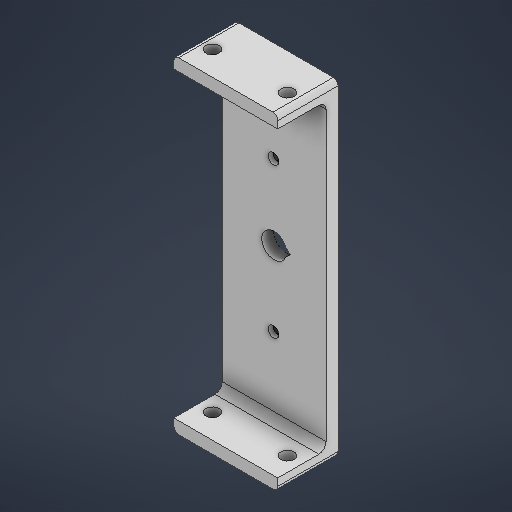
# Autodesk Inventor part: motor_holder
Saved by Autodesk Inventor 2026 (Build 300175050, 175E)
## iProperties
Created: 2025-01-16
Part Number: motor_holder
Material: Generic
Document SubType Name: Modeling
Designer: aduwa
Density: 1 g/cm^3
Appearance: Default
Author: aduwa
Autodesk Inventor part; units mm, degrees
ref_plane "YZ Plane" through (0, 0, 0) normal (1, 0, 0) x (0, 1, 0)
ref_plane "XZ Plane" through (0, 0, 0) normal (0, 1, 0) x (-1, 0, 0)
ref_plane "XY Plane" through (0, 0, 0) normal (0, 0, 1) x (1, 0, 0)
sketch "Sketch1" plane through (0, 0, 0) normal (0, 0, 1) x (1, 0, 0)
  circle A0 centre (0, 0) radius 2.25
  circle A1 centre (31, 0) radius 2.25
  circle A2 centre (0, 31) radius 2.25
  circle A3 centre (31, 31) radius 2.25
  circle A4 centre (15.5, 15.5) radius 5.125
  line L0 (-6, 37) -> (37, 37)
  line L1 (37, 37) -> (37, -6)
  line L2 (37, -6) -> (-6, -6)
  line L3 (-6, -6) -> (-6, 37)
  line L4 (-6, 37) -> (37, -6) construction
  line L5 (37, 37) -> (-6, -6) construction
  line L6 (-6, -6) -> (37, -6)
  line L7 (37, -6) -> (37, -52)
  line L8 (37, -52) -> (-6, -52)
  line L9 (-6, -52) -> (-6, -6)
  line L10 (-6, 15.5) -> (0, 15.5)
  line L11 (37, 37) -> (37, 83)
  line L12 (37, 83) -> (-6, 83)
  line L13 (-6, 83) -> (-6, 37)
  line L14 (20.625, 15.5) -> (22.125, 15.5)
  line L15 (22.125, 15.5) -> (20.2868, 17.3309)
  line L16 (22.125, 15.5) -> (20.2868, 13.6691)
  point P0 (37, 37)
  dimension "d3" = 4.5
  dimension "d5" = 31
  dimension "d6" = 10.25
  dimension "d7" = 43
  dimension "d8" = 43
  dimension "d9" = 67.5
  dimension "d10" = 31
  dimension "d44" = 1.5
  constraints: 34 end point, 5 centre point, 4 horizontal, 4 parallel, 3 equal radius, 3 midpoint, 3 point on circle, 3 symmetric about line, 2 perpendicular, 2 vertical alignment, 1 horizontal alignment
  measures "d3" diameter of A0
  measures "d5" distance of A0.centre A2.centre
  measures "d6" diameter of A4
  measures "d7" distance of L1.end L2.end
  measures "d8" distance of L0.end L1.end
  measures "d9" distance from line of L8 A4.centre
  measures "d10" distance of A3.centre A2.centre
  measures "d44" distance of L14.start L14.end
extrude "Extrusion1" add sketch "Sketch1" against normal blind 5 contours A0 | A1 | A2 | A3 | L13 L12 L11 L0 | L0 L1 L2 L3 | L7 L8 L9 L2
sketch "Sketch2" plane through (0, 0, 0) normal (0, 0, 1) x (1, 0, 0)
  line L0 (37, -52) -> (-6, -52) projected
  line L1 (37, 83) -> (37, -52) projected
  line L2 (-6, -52) -> (37, -52)
  line L3 (37, -52) -> (37, -47)
  line L4 (37, -47) -> (-6, -47)
  line L5 (-6, -47) -> (-6, -52)
  line L6 (-6, 15.5) -> (0, 15.5) projected
  line L7 (37, 78) -> (-6, 78)
  line L8 (-6, 78) -> (37, 78)
  line L9 (-6, 83) -> (-6, -52) projected
  line L10 (-6, -52) -> (37, -52) projected
  line L11 (37, -52) -> (37, 83) projected
  line L12 (37, 83) -> (-6, 83) projected
  arc A0 (20.2868, 17.3309) -> (20.2868, 13.6691) centre (15.5, 15.5) ccw projected
  line L13 (22.125, 15.5) -> (20.2868, 13.6691) projected
  line L14 (20.2868, 17.3309) -> (22.125, 15.5) projected
  point P0 (0, 0)
  point P1 (37, 37)
  point P2 (-6, 37)
  point P3 (-6, 78)
  point P4 (37, 78)
  dimension "d13" = 5
  constraints: 12 end point, 3 equal length, 2 symmetric about line, 1 horizontal, 1 perpendicular, 1 point on line
  measures "d13" distance of L3.end L2.end
extrude "Extrusion2" add sketch "Sketch2" along normal blind 20 contours L0 L5 L4 L1 | L7 L9 L12 L1
sketch "Sketch3" plane through (-6, -47, 0) normal (0, 1, 0) x (1, 0, 0)
  circle A0 centre (6, -10) radius 2.75
  circle A1 centre (37, -10) radius 2.75
  line L0 (0, 5) -> (0, -20) projected
  line L1 (0, 0) -> (0, -20) projected
  line L2 (43, 0) -> (43, -20) projected
  line L3 (0, 5) -> (43, 5) projected
  line L4 (0, 0) -> (43, 0) projected
  line L5 (43, 5) -> (0, 5) projected
  line L6 (6, -10) -> (6, -15) construction
  arc A2 (8.75, -10) -> (3.25, -10) centre (6, -10) ccw
  line L7 (21.5, 0) -> (21.5, -10)
  arc A3 (39.75, -10) -> (34.25, -10) centre (37, -10) ccw
  line L8 (6, -10) -> (6, -5) construction
  line L9 (3.25, -10) -> (3.25, -5)
  line L10 (8.75, -5) -> (8.75, -10)
  arc A4 (3.25, -10) -> (8.75, -10) centre (6, -10) ccw
  arc A5 (8.75, -5) -> (3.25, -5) centre (6, -5) ccw
  line L11 (37, -10) -> (37, -5) construction
  line L12 (39.75, -10) -> (39.75, -5)
  line L13 (34.25, -5) -> (34.25, -10)
  arc A6 (39.75, -5) -> (34.25, -5) centre (37, -5) ccw
  point P0 (6, 0)
  point P1 (0, -10)
  point P2 (6, -12.5)
  point P3 (6, -7.5)
  point P4 (39.75, -10)
  point P5 (3.25, -10)
  dimension "d16" = 5.5
  dimension "d17" = 31
  dimension "d23" = 6
  dimension "d38" = 15
  dimension "d39" = 5
  dimension "d43" = 5
  constraints: 22 end point, 10 point on circle, 9 symmetric about line, 7 centre point, 4 midpoint, 4 tangent, 3 equal radius, 3 vertical, 1 horizontal alignment, 1 parallel, 2 other
  measures "d16" diameter of A0
  measures "d17" distance of A1.centre L6.start
  measures "d23" distance from line of L0 L6.start
  measures "d38" distance from line of L5 L6.start
  measures "d39" distance of L6.start L6.end
  measures "d43" distance of L6.start L8.end
extrude "Extrusion3" [suppressed]
sketch "Sketch8" plane through (-6, 83, 0) normal (0, -1, 0) x (1, 0, 0)
  circle A0 centre (6, 10) radius 2.75 projected
  circle A1 centre (37, 10) radius 2.75 projected
  point P0 (6, 0)
extrude "Extrusion8" cut sketch "Sketch8" along normal blind 160.5
fillet "Fillet2" [suppressed]
sketch "Sketch9" plane through (0, 0, -5) normal (0, 0, -1) x (-1, 0, 0)
  circle A0 centre (-15.235, 46.5) radius 2.25
  circle A1 centre (-15.235, -15.5) radius 2.25
  line L0 (-37, 83) -> (-37, -52) projected
  line L1 (-37, -52) -> (6, -52) projected
  line L2 (6, -52) -> (6, 83) projected
  line L3 (6, 83) -> (-37, 83) projected
  arc A2 (-20.2868, 13.6691) -> (-20.2868, 17.3309) centre (-15.5, 15.5) ccw projected
  line L4 (-20.2868, 13.6691) -> (-22.125, 15.5) projected
  line L5 (-22.125, 15.5) -> (-20.2868, 17.3309) projected
  point P0 (0, 0)
  dimension "d45" = 62
  dimension "d46" = 31
  dimension "d49" = 4.5
  constraints: 2 centre point, 1 equal radius, 1 vertical alignment
  measures "d45" distance of A1.centre A0.centre
  measures "d46" vertical distance of A2.centre A0.centre
  measures "d49" diameter of A0
extrude "Extrusion9" cut sketch "Sketch9" against normal blind 10 contours A0 | A1
sketch "Sketch10" plane through (0, 0, -5) normal (0, 0, 1) x (1, 0, 0)
  circle A0 centre (15.235, -15.5) radius 2.25 projected
  circle A1 centre (15.235, 46.5) radius 2.25 projected
  line L0 (-6, -47) -> (37, -47) projected
  line L1 (37, -47) -> (37, 78) projected
  line L2 (37, 78) -> (-6, 78) projected
  line L3 (-6, 78) -> (-6, -47) projected
  arc A2 (20.2868, 17.3309) -> (20.2868, 13.6691) centre (15.5, 15.5) ccw projected
  line L4 (11.286, 46.5) -> (13.2605, 49.92)
  line L5 (13.2605, 49.92) -> (17.2096, 49.92)
  line L6 (17.2096, 49.92) -> (19.1841, 46.5)
  line L7 (19.1841, 46.5) -> (17.2096, 43.08)
  line L8 (17.2096, 43.08) -> (13.2605, 43.08)
  line L9 (13.2605, 43.08) -> (11.286, 46.5)
  line L10 (10.9973, 46.5) -> (13.1162, 50.17)
  line L11 (13.1162, 50.17) -> (17.3539, 50.17)
  line L12 (17.3539, 50.17) -> (19.4728, 46.5)
  line L13 (19.4728, 46.5) -> (17.3539, 42.83)
  line L14 (17.3539, 42.83) -> (13.1162, 42.83)
  line L15 (13.1162, 42.83) -> (10.9973, 46.5)
  line L16 (15.5, 15.5) -> (12.1559, 15.5)
  circle A3 centre (15.235, -15.5) radius 2.25
  line L17 (11.286, -15.5) -> (13.2605, -18.92)
  line L18 (13.2605, -18.92) -> (17.2096, -18.92)
  line L19 (17.2096, -18.92) -> (19.1841, -15.5)
  line L20 (19.1841, -15.5) -> (17.2096, -12.08)
  line L21 (17.2096, -12.08) -> (13.2605, -12.08)
  line L22 (13.2605, -12.08) -> (11.286, -15.5)
  line L23 (10.9973, -15.5) -> (13.1162, -19.17)
  line L24 (13.1162, -19.17) -> (17.3539, -19.17)
  line L25 (17.3539, -19.17) -> (19.4728, -15.5)
  line L26 (19.4728, -15.5) -> (17.3539, -11.83)
  line L27 (17.3539, -11.83) -> (13.1162, -11.83)
  line L28 (13.1162, -11.83) -> (10.9973, -15.5)
  line L29 (22.125, 15.5) -> (20.2868, 13.6691) projected
  line L30 (20.2868, 17.3309) -> (22.125, 15.5) projected
  point P0 (0, 0)
  dimension "d50" = 6.84
  dimension "d51" = 0.25
  constraints: 50 end point, 14 symmetric about line, 2 coincident, 1 centre point, 1 horizontal, 19 other
  measures "d50" distance between parallel lines of L5 L8
  measures "d51" distance between parallel lines of L9 L15
extrude "M4_hex_neg" cut sketch "Sketch10" along normal blind 3 contours A0 | A1 | L4 L5 L6 L7 L8 L9 | L10 L11 L12 L13 L14 L15 | L22 L21 L20 L19 L18 L17 | L28 L27 L26 L25 L24 L23
fillet "Fillet3" radius 3 2 edges at (15.5, 78, 0) (15.5, -47, 0)
fillet "Fillet4" radius 2 4 edges at (37, -52, 7.5) (37, 83, 7.5) (-6, 83, 7.5) (-6, -52, 7.5)
body "Solid1"
